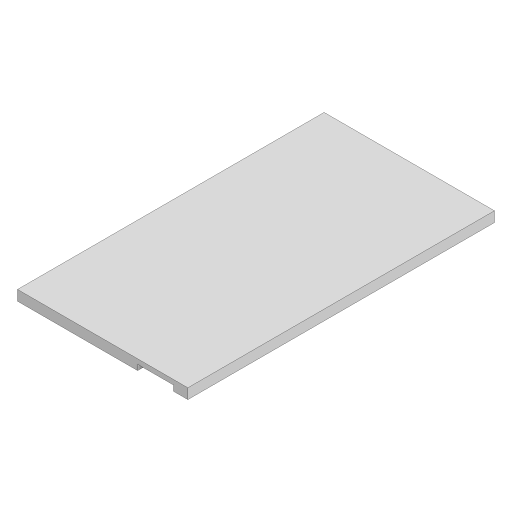
# Autodesk Inventor part: caja_attiny
Saved by Autodesk Inventor 2024 (Build 280153000, 153)
## iProperties
Created: 2023-07-03
Part Number: caja_attiny
Material: Generic
Document SubType Name: Modeling
Designer: ferna
Density: 1 g/cm^3
Appearance: Default
Author: ferna
Autodesk Inventor part; units mm, degrees
ref_plane "YZ Plane" through (0, 0, 0) normal (1, 0, 0) x (0, 1, 0)
ref_plane "XZ Plane" through (0, 0, 0) normal (0, 1, 0) x (-1, 0, 0)
ref_plane "XY Plane" through (0, 0, 0) normal (0, 0, 1) x (1, 0, 0)
sketch "Sketch1" plane through (0, 0, 0) normal (0, 1, 0) x (-1, 0, 0)
  line L0 (0, 0) -> (100, 0)
  line L1 (100, 0) -> (100, -180)
  line L2 (100, -180) -> (0, -180)
  line L3 (0, -180) -> (0, 0)
  dimension "d0" = 100
  dimension "d1" = 180
  constraints: 8 end point, 2 parallel, 1 horizontal, 1 perpendicular
  measures "d0" distance of L1.end L2.end
  measures "d1" distance of L0.end L1.end
extrude "Extrusion1" add sketch "Sketch1" along normal blind 4
sketch "Sketch2" plane through (0, 4, 0) normal (0, 1, 0) x (1, 0, 0)
  line L0 (-100, 180) -> (-100, 0) projected
  line L1 (0, 180) -> (-100, 180) projected
  line L2 (-100, 0) -> (-96, 0)
  line L3 (-96, 0) -> (-96, 180)
  line L4 (-96, 180) -> (-100, 180)
  line L5 (-100, 180) -> (-100, 0)
  line L6 (0, 180) -> (-4, 180)
  line L7 (-4, 180) -> (-4, 0)
  line L8 (-4, 0) -> (0, 0)
  line L9 (0, 0) -> (0, 180)
  dimension "d4" = 4
  dimension "d5" = 4
  constraints: 16 end point, 4 parallel, 2 horizontal, 2 perpendicular, 2 point on line
  measures "d4" distance of L4.end L3.end
  measures "d5" distance of L8.end L7.end
extrude "Extrusion2" add sketch "Sketch2" along normal blind 5 contours L1 L9 L8 L7
sketch "Sketch3" plane through (0, 4, 0) normal (0, 1, 0) x (1, 0, 0)
  line L0 (-4, 180) -> (-4, 0) projected
  line L1 (-4, 0) -> (-34, 0)
  line L2 (-34, 0) -> (-34, 4)
  line L3 (-34, 4) -> (-4, 4)
  line L4 (-4, 4) -> (-4, 0)
  line L5 (-4, 180) -> (-100, 180) projected
  line L6 (-4, 180) -> (-34, 180)
  line L7 (-34, 180) -> (-34, 176)
  line L8 (-34, 176) -> (-4, 176)
  line L9 (-4, 176) -> (-4, 180)
  line L10 (-100, 0) -> (0, 0) projected
  line L11 (-100, 0) -> (-96, 0)
  line L12 (-96, 0) -> (-96, 180)
  line L13 (-96, 180) -> (-100, 180)
  line L14 (-100, 180) -> (-100, 0)
  point P0 (-4, 176)
  point P1 (-4, 4)
  dimension "d8" = 30
  dimension "d9" = 4
  dimension "d10" = 4
  dimension "d11" = 4
  constraints: 24 end point, 6 parallel, 3 horizontal, 3 perpendicular, 1 point on line
  measures "d8" distance of L2.end L3.end
  measures "d9" distance of L1.end L2.end
  measures "d10" distance of L7.end L6.end
  measures "d11" distance of L13.end L12.end
extrude "Extrusion3" add sketch "Sketch3" along normal blind 25 contours L0 L8 L7 L5 | L0 L1 L2 L3 | L12 L10 L14 L5
sketch "Sketch4" plane through (0, 29, 0) normal (0, 1, 0) x (1, 0, 0)
  line L0 (-100, 0) -> (-96, 0) projected
  line L1 (-96, 0) -> (-96, 180) projected
  line L2 (-96, 180) -> (-100, 180) projected
  line L3 (-100, 180) -> (-100, 0) projected
  line L4 (-4, 176) -> (-4, 180) projected
  line L5 (-4, 180) -> (-34, 180) projected
  line L6 (-34, 180) -> (-34, 176) projected
  line L7 (-34, 176) -> (-4, 176) projected
  line L8 (-34, 0) -> (-4, 0) projected
  line L9 (-34, 4) -> (-34, 0) projected
  line L10 (-34, 0) -> (-4, 0) projected
  line L11 (-4, 0) -> (-4, 4) projected
  line L12 (-4, 4) -> (-34, 4) projected
  line L13 (-100, 90) -> (-100, 145)
  line L14 (-100, 145) -> (-96, 145)
  line L15 (-96, 145) -> (-96, 35)
  line L16 (-96, 0) -> (-96, 180) projected
  line L17 (-96, 35) -> (-100, 35)
  line L18 (-100, 35) -> (-100, 90)
  line L19 (-4, 176) -> (-34, 176) projected
  line L20 (-19, 176) -> (-29, 176)
  line L21 (-29, 176) -> (-29, 180)
  line L22 (-29, 180) -> (-9, 180)
  line L23 (0, 180) -> (-100, 180) projected
  line L24 (-9, 180) -> (-9, 176)
  line L25 (-19, 176) -> (-9, 176)
  line L26 (-19, 4) -> (-29, 4)
  line L27 (-29, 4) -> (-29, 0)
  line L28 (-29, 0) -> (-9, 0)
  line L29 (-9, 0) -> (-9, 4)
  line L30 (-4, 4) -> (-34, 4) projected
  line L31 (-9, 4) -> (-19, 4)
  point P0 (0, 0)
  dimension "d14" = 55
  dimension "d15" = 110
  dimension "d16" = 10
  dimension "d17" = 20
  constraints: 30 end point, 16 point on line, 5 perpendicular, 3 midpoint, 2 collinear
  measures "d14" distance of L13.start L13.end
  measures "d15" distance of L14.end L15.end
  measures "d16" distance of L20.start L20.end
  measures "d17" distance of L21.end L22.end
extrude "Extrusion4" add sketch "Sketch4" along normal blind 3 contours L3 L14 L1 L17 | L5 L24 L7 L21 | L27 L12 L29 L8
sketch "Sketch5" plane through (0, 0, 0) normal (0, -1, 0) x (1, 0, 0)
  line L0 (-9, -4) -> (-29, -4) projected
  line L1 (-29, -4) -> (-29, 0) projected
  line L2 (-29, 0) -> (-9, 0) projected
  line L3 (-9, 0) -> (-9, -4) projected
  line L4 (-9, -180) -> (-29, -180) projected
  line L5 (-29, -180) -> (-29, -176) projected
  line L6 (-29, -176) -> (-9, -176) projected
  line L7 (-9, -176) -> (-9, -180) projected
  line L8 (-96, -35) -> (-96, -145) projected
  line L9 (-96, -145) -> (-100, -145) projected
  line L10 (-100, -145) -> (-100, -35) projected
  line L11 (-100, -35) -> (-96, -35) projected
  line L12 (-96, -180) -> (-96, 0) projected
  line L13 (-100, -35) -> (-96, -35)
  line L14 (-96, -35) -> (-96, -34.5)
  line L15 (-96, -34.5) -> (-100, -34.5)
  line L16 (-100, -34.5) -> (-100, -35)
  line L17 (-100, -145) -> (-96, -145)
  line L18 (-96, -145) -> (-96, -145.5)
  line L19 (-96, -145.5) -> (-100, -145.5)
  line L20 (-100, -145.5) -> (-100, -145)
  line L21 (-4, -176) -> (-34, -176) projected
  line L22 (-29, -180) -> (-29.5, -180)
  line L23 (-29.5, -180) -> (-29.5, -176)
  line L24 (-29.5, -176) -> (-29, -176)
  line L25 (-29, -176) -> (-29, -180)
  line L26 (-9, -176) -> (-8.5, -176)
  line L27 (-8.5, -176) -> (-8.5, -180)
  line L28 (-8.5, -180) -> (-9, -180)
  line L29 (-9, -180) -> (-9, -176)
  line L30 (-34, -4) -> (-4, -4) projected
  line L31 (-29, 0) -> (-29.5, 0)
  line L32 (-29.5, 0) -> (-29.5, -4)
  line L33 (-29.5, -4) -> (-29, -4)
  line L34 (-29, -4) -> (-29, 0)
  line L35 (-9, 0) -> (-8.5, 0)
  line L36 (-8.5, 0) -> (-8.5, -4)
  line L37 (-8.5, -4) -> (-9, -4)
  line L38 (-9, -4) -> (-9, 0)
  point P0 (0, 0)
  dimension "d22" = 0.5
  dimension "d23" = 0.5
  dimension "d24" = 0.5
  dimension "d25" = 0.5
  dimension "d26" = 0.5
  dimension "d27" = 0.5
  constraints: 48 end point, 12 parallel, 6 horizontal, 6 perpendicular, 6 point on line
  measures "d22" distance of L14.end L13.end
  measures "d23" distance of L17.end L18.end
  measures "d24" distance of L23.end L24.end
  measures "d25" distance of L27.end L28.end
  measures "d26" distance of L33.end L32.end
  measures "d27" distance of L36.end L37.end
extrude "Extrusion5" cut sketch "Sketch5" against normal blind 3.2
sketch "Sketch6" plane through (0, 32, 0) normal (0, 1, 0) x (1, 0, 0)
  line L0 (-126.3586, 197.6117) -> (20.3273, 197.6117)
  line L1 (20.3273, 197.6117) -> (20.3273, -20.388)
  line L2 (20.3273, -20.388) -> (-126.3586, -20.388)
  line L3 (-126.3586, -20.388) -> (-126.3586, 197.6117)
  point P0 (0, 0)
  constraints: 8 end point, 2 parallel, 1 horizontal, 1 perpendicular
extrude "Extrusion6" cut sketch "Sketch6" against normal up to surface (28 mm away)
sketch "Sketch7" plane through (0, 4, 0) normal (0, 1, 0) x (1, 0, 0)
  line L0 (0, 180) -> (-100, 180) projected
  line L1 (-100, 0) -> (-100, 180) projected
  line L2 (-100, 0) -> (0, 0) projected
  line L3 (0, 180) -> (0, 0) projected
extrude "Extrusion7" add sketch "Sketch7" along normal blind 2
body "Solid1"
